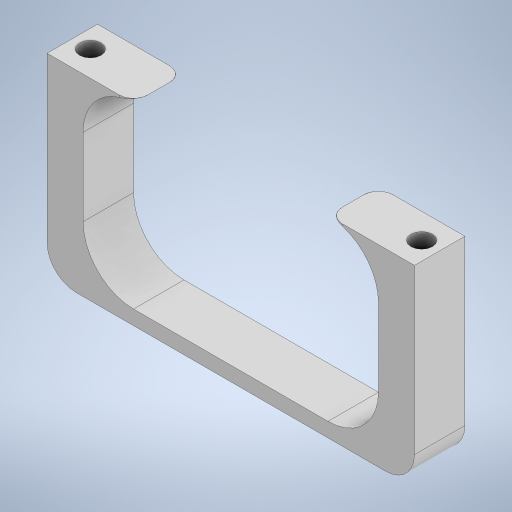
# Autodesk Inventor part: Clamp_v4_bot
Saved by Autodesk Inventor 2024.3 (Build 283343000, 343)
## iProperties
Created: 2024-04-15
Part Number: Clamp_v4_bot
Material: Generic
Document SubType Name: Modeling
Designer: magn1
Density: 1 g/cm^3
Appearance: Default
Author: magn1
Autodesk Inventor part; units mm, degrees
ref_plane "YZ Plane" through (0, 0, 0) normal (1, 0, 0) x (0, 1, 0)
ref_plane "XZ Plane" through (0, 0, 0) normal (0, 1, 0) x (-1, 0, 0)
ref_plane "XY Plane" through (0, 0, 0) normal (0, 0, 1) x (1, 0, 0)
sketch "Sketch1" plane through (0, 0, 0) normal (0, 0, 1) x (1, 0, 0)
  line L0 (17, -8.875) -> (-17, -8.875) construction
  line L1 (-17, -8.875) -> (-17, 8.875) construction
  line L2 (-17, 8.875) -> (17, 8.875) construction
  line L3 (17, 8.875) -> (17, -8.875) construction
  line L4 (17, -8.875) -> (-17, 8.875) construction
  line L5 (-17, -8.875) -> (17, 8.875) construction
  line L6 (20.5, 12.375) -> (-20.5, 12.375)
  line L7 (-20.5, 12.375) -> (-20.5, -12.375)
  line L8 (-20.5, -12.375) -> (20.5, -12.375)
  line L9 (20.5, -12.375) -> (20.5, 12.375)
  line L10 (20.5, 12.375) -> (-20.5, -12.375) construction
  line L11 (-20.5, 12.375) -> (20.5, -12.375) construction
  line L12 (-25.5, -14.375) -> (25.5, -14.375)
  line L13 (25.5, -14.375) -> (25.5, 14.375)
  line L14 (25.5, 14.375) -> (-25.5, 14.375)
  line L15 (-25.5, 14.375) -> (-25.5, -14.375)
  line L16 (-25.5, -14.375) -> (25.5, 14.375) construction
  line L17 (25.5, -14.375) -> (-25.5, 14.375) construction
  line L18 (-20.5, 12.375) -> (-25.5, 12.375)
  line L19 (20.5, 12.375) -> (25.5, 12.375)
  point P0 (0, 0)
  dimension "d0" = 34
  dimension "d1" = 17.75
  dimension "d2" = 41
  dimension "d3" = 24.75
  dimension "d4" = 51
  dimension "d5" = 28.75
  constraints: 40 end point, 6 midpoint, 6 parallel, 4 perpendicular, 3 horizontal, 3 point on line
  measures "d0" distance of L1.end L2.end
  measures "d1" distance of L0.end L1.end
  measures "d2" distance of L8.end L7.end
  measures "d3" distance of L7.end L6.end
  measures "d4" distance of L14.end L13.end
  measures "d5" distance of L13.end L12.end
extrude "Extrusion1" add sketch "Sketch1" along normal blind 7 contours L19 L13 L12 L15 L18 L7 L8 L9
sketch "Sketch3" plane through (-25.5, 12.375, 0) normal (0, 1, 0) x (1, 0, 0)
  line L0 (0, 0) -> (0, -7) construction
  line L1 (0, -3.5) -> (2.5, -3.5) construction
  line L2 (51, 0) -> (51, -7) construction
  line L3 (51, -3.5) -> (48.5, -3.5) construction
  circle A0 centre (2.5, -3.5) radius 1.5
  circle A1 centre (48.5, -3.5) radius 1.5
  point P0 (25.5, 0)
  dimension "d18" = 2.5
  dimension "d19" = 2.5
  dimension "d20" = 3
  dimension "d21" = 3
  constraints: 4 end point, 2 centre point, 2 coincident, 2 horizontal, 2 midpoint
  measures "d18" distance of L1.start L1.end
  measures "d19" distance of L3.start L3.end
  measures "d20" diameter of A0
  measures "d21" diameter of A1
extrude "Extrusion3" cut sketch "Sketch3" against normal blind 7
fillet "Fillet1" radius 7 2 edges at (-20.5, -12.375, 3.5) (20.5, -12.375, 3.5)
fillet "Fillet2" radius 4 2 edges at (-25.5, -14.375, 3.5) (25.5, -14.375, 3.5)
sketch "Sketch4" plane through (0, 0, 7) normal (0, 0, 1) x (1, 0, 0)
  line L0 (-20.5, 12.375) -> (-25.5, 12.375) construction
  line L1 (-20.5, 12.375) -> (-20.5, 10.375) construction
  line L2 (-20.5, -5.375) -> (-20.5, 12.375) construction
  line L3 (-20.5, 12.375) -> (-18.5, 12.375) construction
  line L4 (-18.5, 12.375) -> (-16.5, 12.375) construction
  line L5 (-20.5, 10.375) -> (-13.5, 10.375) construction
  line L6 (-13.5, 12.375) -> (-13.5, 5.375) construction
  circle A0 centre (-13.5, 5.375) radius 7
  line L7 (-20.5, 12.375) -> (-13.5, 12.375)
  line L8 (-20.5, 5.375) -> (-20.5, 12.375)
  point P0 (0, 0)
  dimension "d27" = 2
  dimension "d28" = 90
  dimension "d31" = 7
  dimension "d32" = 7
  dimension "d33" = 7
  constraints: 14 end point, 4 horizontal, 2 collinear, 2 point on circle, 2 point on line, 1 centre point, 1 coincident, 1 perpendicular, 1 vertical
  measures "d27" distance of L0.start L1.end
  measures "d28" angle of L1 L3
  measures "d31" distance of L1.end L5.end
  measures "d32" distance of L6.start L6.end
  measures "d33" distance from line of L2 L6.start
extrude "Extrusion4" add sketch "Sketch4" against normal up to surface (7 mm away) contours A0 L8 L7
mirror "Mirror1" about plane through (0, 0, 0) normal (1, 0, 0) of "Extrusion4"
sketch "Sketch5" plane through (-25.5, 12.375, 7) normal (0, 1, 0) x (1, 0, 0)
  line L0 (0, 7) -> (0, 0) construction
  line L1 (12, 0) -> (0, 0) construction
  line L2 (0, 7) -> (10, 7) construction
  line L3 (12, 5) -> (12, 2) construction
  line L4 (10, 0) -> (0, 0) construction
  line L5 (0, 0) -> (0, 7) construction
  arc A0 (12, 5) -> (10, 7) centre (10, 5) ccw
  arc A1 (10, 0) -> (12, 2) centre (10, 2) ccw
  line L6 (12, 5) -> (12, 2)
  line L7 (10, 0) -> (0, 0)
  line L8 (0, 7) -> (0, 0)
  line L9 (0, 7) -> (10, 7)
  line L10 (39, 7) -> (39, 0) construction
  line L11 (51, 0) -> (39, 0) construction
  line L12 (41, 7) -> (51, 7) construction
  line L13 (51, 7) -> (51, 0) construction
  line L14 (51, 0) -> (41, 0) construction
  line L15 (39, 2) -> (39, 5) construction
  arc A2 (41, 7) -> (39, 5) centre (41, 5) ccw
  arc A3 (39, 2) -> (41, 0) centre (41, 2) ccw
  line L16 (41, 7) -> (51, 7)
  line L17 (51, 0) -> (51, 7)
  line L18 (51, 0) -> (41, 0)
  line L19 (39, 2) -> (39, 5)
  line L20 (12, 0) -> (12, 7) projected
  line L21 (10, 7) -> (12, 7)
  line L22 (12, 7) -> (12, 5)
  line L23 (12, 2) -> (12, 0)
  line L24 (12, 0) -> (10, 0)
  line L25 (41, 7) -> (39, 7)
  line L26 (39, 5) -> (39, 7)
  line L27 (39, 2) -> (39, 0)
  line L28 (41, 0) -> (39, 0)
  point P0 (25.5, 7)
  dimension "d36" = 2
  dimension "d37" = 2
  dimension "d38" = 2
  constraints: 48 end point, 12 tangent, 9 perpendicular, 8 point on circle, 5 collinear, 4 centre point, 4 horizontal, 4 parallel, 4 point on line, 2 vertical, 1 equal radius
  measures "d36" radius of A0
  measures "d37" radius of A1
  measures "d38" radius of A2
extrude "Extrusion5" cut sketch "Sketch5" against normal blind 1 contours A0 L21 L20 | L20 L24 A1 | A2 L26 L25 | A3 L28 L27
body "Solid1"
